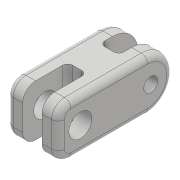
# Autodesk Inventor part: Link_Tensionador
Saved by Autodesk Inventor 2018 (Build 220112000, 112)
## iProperties
Created: 2021-04-29
Part Number: Link_Tensionador
Material: Generic
Document SubType Name: Modeling
Designer: l01767
Density: 1 g/cm^3
Appearance: Default
Author: l01767
Autodesk Inventor part; units mm, degrees
ref_plane "YZ Plane" through (0, 0, 0) normal (1, 0, 0) x (0, 1, 0)
ref_plane "XZ Plane" through (0, 0, 0) normal (0, 1, 0) x (-1, 0, 0)
ref_plane "XY Plane" through (0, 0, 0) normal (0, 0, 1) x (1, 0, 0)
sketch "Sketch1" plane through (0, 0, 0) normal (1, 0, 0) x (0, 1, 0)
  line L0 (-70, 40) -> (50, 40)
  line L1 (90, 0) -> (90, 0)
  line L2 (50, -40) -> (-70, -40)
  line L3 (-90, -20) -> (-90, 20)
  line L4 (-90, 40) -> (90, -40) construction
  line L5 (90, 40) -> (-90, -40) construction
  circle A0 centre (55, 0) radius 11
  line L6 (0, 0) -> (0, -40.3764)
  circle A1 centre (-55, 0) radius 18
  arc A2 (90, 0) -> (50, 40) centre (50, 0) ccw
  arc A3 (50, -40) -> (90, 0) centre (50, 0) ccw
  arc A4 (-70, 40) -> (-90, 20) centre (-70, 20) ccw
  arc A5 (-90, -20) -> (-70, -40) centre (-70, -20) ccw
  dimension "d0" = 180
  dimension "d1" = 22
  dimension "d2" = 36
  dimension "d3" = 110
  dimension "d4" = 80
  dimension "d5" = 40
  dimension "d6" = 20
  constraints: 14 end point, 8 point on circle, 8 point on line, 8 tangent, 6 centre point, 2 midpoint, 2 parallel, 1 concentric, 1 equal radius, 1 horizontal, 1 horizontal alignment, 1 perpendicular, 1 symmetric about line, 1 vertical
  measures "d0" distance of L4.end L5.end
  measures "d1" diameter of A0
  measures "d2" diameter of A1
  measures "d3" distance of A1.centre A0.centre
  measures "d4" distance of L5.start L4.end
  measures "d5" radius of A2
  measures "d6" radius of A4
extrude "Extrusion1" add sketch "Sketch1" along normal mid plane 80
fillet "Fillet1" radius 10 12 edges at (40, -84.1421, 34.1421) (40, -90, 0) (40, -84.1421, -34.1421) (40, -10, -40) (40, 78.2843, 28.2843) (40, -10, 40) (-40, 78.2843, -28.2843) (-40, -10, -40) (-40, -84.1421, -34.1421) (-40, -90, 0) (-40, -84.1421, 34.1421) (-40, -10, 40)
sketch "Sketch2" plane through (-30, -70, 40) normal (0, 0, 1) x (1, 0, 0)
  line L0 (0, 160) -> (60, 160) projected
  line L1 (15, 160) -> (45, 160)
  line L2 (45, 160) -> (45, 100)
  line L3 (45, 100) -> (15, 100)
  line L4 (15, 100) -> (15, 160)
  line L5 (15, -20) -> (45, -20)
  line L6 (45, -20) -> (45, 50)
  line L7 (45, 50) -> (15, 50)
  line L8 (15, 50) -> (15, -20)
  line L9 (0, -20) -> (60, -20) projected
  line L10 (30, 160) -> (30, 100) construction
  point P0 (30, 70)
  dimension "d10" = 60
  dimension "d11" = 70
  dimension "d12" = 30
  constraints: 18 end point, 4 parallel, 3 point on line, 2 horizontal, 2 midpoint, 2 perpendicular, 1 collinear, 1 vertical alignment
  measures "d10" distance of L1.end L2.end
  measures "d11" distance of L5.end L6.end
  measures "d12" distance of L2.end L3.end
extrude "Extrusion2" cut sketch "Sketch2" against normal through all
fillet "Fillet2" radius 8 4 edges at (-15, 30, 0) (15, 30, 0) (-15, -20, 0) (15, -20, 0)
equation "\"d5\" = 0.5 * d4"
body "Solid1"
